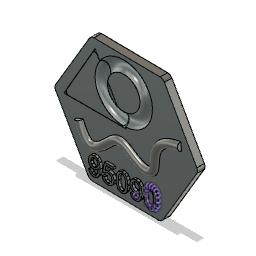
medallion with 95090 Torus Snake v3 (Autodesk Fusion 360 design; units mm, degrees)
Autodesk Fusion 360 part; units mm, degrees
note: some values were not read from the file. Set by a fixed rule: which sketch regions a step uses.
sketch "Sketch1" plane through (0, 0, 0) normal (0, 0, 1) x (1, 0, 0)
  line L0 (13.5687, 24.844) -> (-12.9876, 25.1527)
  line L1 (-14.7311, 24.1729) -> (-28.2766, 1.3288)
  line L2 (-28.2999, -0.6711) -> (-15.2891, -23.8239)
  line L3 (-13.5687, -24.844) -> (12.9876, -25.1527)
  line L4 (14.7311, -24.1729) -> (28.2766, -1.3288)
  line L5 (28.2999, 0.6711) -> (15.2891, 23.8239)
  arc A0 (-12.9876, 25.1527) -> (-14.7311, 24.1729) centre (-13.0108, 23.1528) ccw
  arc A1 (15.2891, 23.8239) -> (13.5687, 24.844) centre (13.5455, 22.8441) ccw
  arc A2 (28.2766, -1.3288) -> (28.2999, 0.6711) centre (26.5563, -0.3087) ccw
  arc A3 (12.9876, -25.1527) -> (14.7311, -24.1729) centre (13.0108, -23.1528) ccw
  arc A4 (-15.2891, -23.8239) -> (-13.5687, -24.844) centre (-13.5455, -22.8441) ccw
  arc A5 (-28.2766, 1.3288) -> (-28.2999, -0.6711) centre (-26.5563, 0.3087) ccw
  point P0 (-12.5, 7.2169)
  dimension "d1" = 25
  dimension "d7" = 2
  dimension "d8" = 2
  dimension "d9" = 2
  dimension "d10" = 2
  dimension "d11" = 2
  dimension "d12" = 2
  constraint tangent L0 A0
  constraint tangent L1 A0
  constraint tangent L0 A1
  constraint tangent L5 A1
  constraint tangent L4 A2
  constraint tangent L5 A2
  constraint tangent L3 A3
  constraint tangent L4 A3
  constraint tangent L2 A4
  constraint tangent L3 A4
  constraint tangent L1 A5
  constraint tangent L2 A5
  measures "d1" distance of origin L5
  measures "d7" radius of A0
  measures "d8" radius of A1
  measures "d9" radius of A2
  measures "d10" radius of A3
  measures "d11" radius of A4
  measures "d12" radius of A5
extrude "Extrude1" add sketch "Sketch1" along normal blind 3 makes body 1
sketch "Sketch2" plane through (0, 0, 0) normal (0, 0, 1) x (1, 0, 0)
  line L0 (-64.3097, 3.8259) -> (-50.5509, -12.3499)
  line L1 (-48.8472, -12.0378) -> (-41.718, 7.9657)
  line L2 (-42.8402, 9.285) -> (-63.7283, 5.4574)
  arc A0 (-41.718, 7.9657) -> (-42.8402, 9.285) centre (-42.6599, 8.3014) ccw
  arc A1 (-50.5509, -12.3499) -> (-48.8472, -12.0378) centre (-49.7892, -11.702) ccw
  arc A2 (-63.7283, 5.4574) -> (-64.3097, 3.8259) centre (-63.548, 4.4738) ccw
  point P0 (-49.4287, -13.6693)
  point P1 (-41.1365, 9.5972)
  point P2 (-53.3624, 0.343)
  dimension "d15" = 24.7
  dimension "d16" = 1
  dimension "d17" = 1
  dimension "d21" = 60
  dimension "d22" = 60
  dimension "d24" = 1
  constraint coincident P1 L1
  constraint coincident P1 L2
  constraint tangent L1 A0
  constraint tangent L2 A0
  constraint coincident P0 L0
  constraint coincident P0 L1
  constraint tangent L0 A1
  constraint tangent L1 A1
  constraint tangent L0 A2
  constraint tangent L2 A2
  measures "d15" distance of P0 P1
  measures "d16" radius of A0
  measures "d17" radius of A1
  measures "d21" angle of L0 L2
  measures "d22" angle of L0 L1
  measures "d24" radius of A2
extrude "Extrude2" add sketch "Sketch2" along normal blind 3 separate body makes body 2
sketch "Sketch4" plane through (0, 0, 3) normal (0, 0, 1) x (1, 0, 0)
  arc A0 (-28.2766, 1.3288) -> (-28.2999, -0.6711) centre (-26.5563, 0.3087) ccw
  line L0 (-28.2999, -0.6711) -> (-15.2891, -23.8239)
  arc A1 (-15.2891, -23.8239) -> (-13.5687, -24.844) centre (-13.5455, -22.8441) ccw
  line L1 (-13.5687, -24.844) -> (12.9876, -25.1527)
  arc A2 (12.9876, -25.1527) -> (14.7311, -24.1729) centre (13.0108, -23.1528) ccw
  line L2 (14.7311, -24.1729) -> (28.2766, -1.3288)
  arc A3 (28.2766, -1.3288) -> (28.2999, 0.6711) centre (26.5563, -0.3087) ccw
  line L3 (28.2999, 0.6711) -> (15.2891, 23.8239)
  arc A4 (15.2891, 23.8239) -> (13.5687, 24.844) centre (13.5455, 22.8441) ccw
  line L4 (13.5687, 24.844) -> (-12.9876, 25.1527)
  arc A5 (-12.9876, 25.1527) -> (-14.7311, 24.1729) centre (-13.0108, 23.1528) ccw
  line L5 (-14.7311, 24.1729) -> (-28.2766, 1.3288)
  line L6 (-12.5, 21.6506) -> (-25, 0)
  line L7 (-25, 0) -> (0, 0)
  line L8 (0, 0) -> (-12.5, 21.6506)
  point P0 (-12.5, 7.2169)
  dimension "d25" = 25
  constraint coincident L7.end L8.start
  constraint horizontal L7
  measures "d25" distance of L6.start L7.end
extrude "Extrude3" cut sketch "Sketch4" against normal up to surface (3 mm away) contours L6 L7 L8 bodies 1
sketch "Sketch5" plane through (0, 0, 3) normal (0, 0, 1) x (1, 0, 0)
  line L0 (-12.5, 21.6506) -> (0, 0)
  line L1 (0, 0) -> (-25, 0)
  line L2 (-25, 0) -> (-12.5, 21.6506)
  arc A0 (-28.2766, 1.3288) -> (-28.2999, -0.6711) centre (-26.5563, 0.3087) ccw
  line L3 (-28.2999, -0.6711) -> (-15.2891, -23.8239)
  arc A1 (-15.2891, -23.8239) -> (-13.5687, -24.844) centre (-13.5455, -22.8441) ccw
  line L4 (-13.5687, -24.844) -> (12.9876, -25.1527)
  arc A2 (12.9876, -25.1527) -> (14.7311, -24.1729) centre (13.0108, -23.1528) ccw
  line L5 (14.7311, -24.1729) -> (28.2766, -1.3288)
  arc A3 (28.2766, -1.3288) -> (28.2999, 0.6711) centre (26.5563, -0.3087) ccw
  line L6 (28.2999, 0.6711) -> (15.2891, 23.8239)
  arc A4 (15.2891, 23.8239) -> (13.5687, 24.844) centre (13.5455, 22.8441) ccw
  line L7 (13.5687, 24.844) -> (-12.9876, 25.1527)
  arc A5 (-12.9876, 25.1527) -> (-14.7311, 24.1729) centre (-13.0108, 23.1528) ccw
  line L8 (-14.7311, 24.1729) -> (-28.2766, 1.3288)
  line L9 (-14.1937, -22.0754) -> (12.7204, -22.0754) construction
  line L10 (12.7204, -22.0754) -> (12.7204, -12.0754) construction
  line L11 (12.7204, -12.0754) -> (-14.1937, -12.0754) construction
  line L12 (-14.1937, -12.0754) -> (-14.1937, -22.0754) construction
  text T0 "95090" font "Arial" height 10 align ink ink in box 0 x 0 at (-14.1837, -22.0554) x (1, 0) y (0, 1) spacing 1 height is em
  constraint perpendicular L9 L10
  constraint parallel L9 L11
  constraint parallel L10 L12
extrude "Extrude4" add sketch "Sketch5" along normal blind 1 text T0 bodies 1
sketch "Sketch6" plane through (0, 0, 3) normal (0, 0, 1) x (1, 0, 0)
  spline S0 degree 3 poles (3.1161, -18.862) (2.9368, -18.6225) (2.5605, -18.1199) (2.5214, -17.4917) (2.5009, -17.1628) knots 0 0 0 0 0.087808 0.184257 0.184257 0.184257 0.184257
  spline S1 degree 3 poles (2.5009, -17.1628) (2.5222, -16.8233) (2.5631, -16.1742) (2.9541, -15.6567) (3.1405, -15.4099) knots 0 0 0 0 0.099559 0.190304 0.190304 0.190304 0.190304
  spline S2 degree 3 poles (3.1405, -15.4099) (3.3707, -15.2162) (3.8369, -14.824) (4.4444, -14.7721) (4.7519, -14.7458) knots 0 0 0 0 0.087967 0.178131 0.178131 0.178131 0.178131
  spline S3 degree 3 poles (4.7519, -14.7458) (4.9791, -14.7612) (5.4319, -14.792) (5.8287, -15.0121) (6.0263, -15.1218) knots 0 0 0 0 0.067431 0.134333 0.134333 0.134333 0.134333
  spline S4 degree 3 poles (6.0263, -15.1218) (6.2093, -15.2633) (6.5846, -15.5535) (6.7966, -15.9783) (6.9052, -16.196) knots 0 0 0 0 0.068468 0.140401 0.140401 0.140401 0.140401
  spline S5 degree 3 poles (6.9052, -16.196) (6.993, -16.4772) (7.1973, -17.1308) (7.2041, -17.8169) (7.2079, -18.2077) knots 0 0 0 0 0.087942 0.2044 0.2044 0.2044 0.2044
  spline S6 degree 3 poles (7.2079, -18.2077) (7.2023, -18.6215) (7.1923, -19.3637) (6.9966, -20.0788) (6.9101, -20.3952) knots 0 0 0 0 0.123516 0.221554 0.221554 0.221554 0.221554
  spline S7 degree 3 poles (6.9101, -20.3952) (6.8034, -20.6457) (6.5995, -21.1249) (6.2081, -21.4672) (6.0214, -21.6306) knots 0 0 0 0 0.080478 0.153934 0.153934 0.153934 0.153934
  spline S8 degree 3 poles (6.0214, -21.6306) (5.8145, -21.7545) (5.3906, -22.0083) (4.8971, -22.0395) (4.6444, -22.0554) knots 0 0 0 0 0.071242 0.145975 0.145975 0.145975 0.145975
  spline S9 degree 3 poles (4.6444, -22.0554) (4.382, -22.04) (3.8811, -22.0107) (3.4687, -21.7267) (3.2724, -21.5915) knots 0 0 0 0 0.07717 0.147318 0.147318 0.147318 0.147318
  spline S10 degree 3 poles (3.2724, -21.5915) (3.1119, -21.4131) (2.7741, -21.0375) (2.6814, -20.5395) (2.6327, -20.2781) knots 0 0 0 0 0.070582 0.148635 0.148635 0.148635 0.148635
  line L0 (2.6327, -20.2781) -> (3.4774, -20.1999)
  spline S11 degree 3 poles (4.664, -21.3327) (4.7929, -21.3262) (5.042, -21.3134) (5.2646, -21.2013) (5.372, -21.1472) knots 0 0 0 0 0.038246 0.07391 0.07391 0.07391 0.07391
  spline S12 degree 3 poles (5.372, -21.1472) (5.47, -21.0801) (5.6666, -20.9453) (5.8053, -20.7514) (5.8749, -20.654) knots 0 0 0 0 0.035331 0.070924 0.070924 0.070924 0.070924
  spline S13 degree 3 poles (5.8749, -20.654) (5.9391, -20.5337) (6.0813, -20.267) (6.1593, -19.9746) (6.2021, -19.8142) knots 0 0 0 0 0.040781 0.090394 0.090394 0.090394 0.090394
  spline S14 degree 3 poles (6.3339, -18.74) (6.3336, -18.7156) (6.3328, -18.6569) (6.3304, -18.5984) (6.329, -18.5642) knots 0 0 0 0 0.007325 0.017586 0.017586 0.017586 0.017586
  spline S15 degree 3 poles (6.329, -18.5642) (6.2317, -18.6984) (6.0337, -18.9714) (5.7504, -19.1546) (5.6064, -19.2478) knots 0 0 0 0 0.049266 0.100244 0.100244 0.100244 0.100244
  spline S16 degree 3 poles (5.6064, -19.2478) (5.4513, -19.3233) (5.1397, -19.4749) (4.7938, -19.496) (4.62, -19.5066) knots 0 0 0 0 0.051186 0.102862 0.102862 0.102862 0.102862
  arc A0 (-28.2766, 1.3288) -> (-28.2999, -0.6711) centre (-26.5563, 0.3087) ccw
  line L1 (-28.2999, -0.6711) -> (-15.2891, -23.8239)
  arc A1 (-15.2891, -23.8239) -> (-13.5687, -24.844) centre (-13.5455, -22.8441) ccw
  line L2 (-13.5687, -24.844) -> (12.9876, -25.1527)
  arc A2 (12.9876, -25.1527) -> (14.7311, -24.1729) centre (13.0108, -23.1528) ccw
  line L3 (14.7311, -24.1729) -> (28.2766, -1.3288)
  arc A3 (28.2766, -1.3288) -> (28.2999, 0.6711) centre (26.5563, -0.3087) ccw
  line L4 (28.2999, 0.6711) -> (15.2891, 23.8239)
  arc A4 (15.2891, 23.8239) -> (13.5687, 24.844) centre (13.5455, 22.8441) ccw
  line L5 (13.5687, 24.844) -> (-12.9876, 25.1527)
  arc A5 (-12.9876, 25.1527) -> (-14.7311, 24.1729) centre (-13.0108, 23.1528) ccw
  line L6 (-14.7311, 24.1729) -> (-28.2766, 1.3288)
  line L7 (-12.5, 21.6506) -> (0, 0)
  line L8 (0, 0) -> (-25, 0)
  line L9 (-25, 0) -> (-12.5, 21.6506)
  line L10 (-8.6222, -20.0583) -> (-7.6993, -19.9802)
  spline S17 degree 3 poles (-7.6993, -19.9802) (-7.6597, -20.1853) (-7.5864, -20.5648) (-7.3392, -20.8601) (-7.2257, -20.9958) knots 0 0 0 0 0.06147 0.113705 0.113705 0.113705 0.113705
  spline S18 degree 3 poles (-7.2257, -20.9958) (-7.093, -21.0941) (-6.8244, -21.293) (-6.4911, -21.3194) (-6.3224, -21.3327) knots 0 0 0 0 0.048487 0.098156 0.098156 0.098156 0.098156
  spline S19 degree 3 poles (-6.3224, -21.3327) (-6.1184, -21.3123) (-5.7079, -21.2711) (-5.4021, -20.9938) (-5.2481, -20.8542) knots 0 0 0 0 0.059802 0.120401 0.120401 0.120401 0.120401
  spline S20 degree 3 poles (-5.2481, -20.8542) (-5.1201, -20.6752) (-4.8492, -20.2965) (-4.8227, -19.8304) (-4.8087, -19.5847) knots 0 0 0 0 0.06469 0.136821 0.136821 0.136821 0.136821
  spline S21 degree 3 poles (-4.8087, -19.5847) (-4.8218, -19.3522) (-4.8465, -18.9133) (-5.1097, -18.5629) (-5.2335, -18.3982) knots 0 0 0 0 0.068094 0.12856 0.12856 0.12856 0.12856
  spline S22 degree 3 poles (-5.2335, -18.3982) (-5.3882, -18.2715) (-5.7087, -18.0089) (-6.1228, -17.9791) (-6.337, -17.9636) knots 0 0 0 0 0.058504 0.12122 0.12122 0.12122 0.12122
  spline S23 degree 3 poles (-6.337, -17.9636) (-6.474, -17.9711) (-6.7425, -17.9857) (-6.9849, -18.102) (-7.1036, -18.1589) knots 0 0 0 0 0.040699 0.079802 0.079802 0.079802 0.079802
  spline S24 degree 3 poles (-7.1036, -18.1589) (-7.2108, -18.2263) (-7.4213, -18.3586) (-7.5685, -18.5587) (-7.6407, -18.657) knots 0 0 0 0 0.037605 0.073834 0.073834 0.073834 0.073834
  line L11 (-7.6407, -18.657) -> (-8.4659, -18.5495)
  line L12 (-8.4659, -18.5495) -> (-7.7726, -14.8728)
  line L13 (-7.7726, -14.8728) -> (-4.213, -14.8728)
  line L14 (-4.213, -14.8728) -> (-4.213, -15.7126)
  line L15 (-4.213, -15.7126) -> (-7.0694, -15.7126)
  line L16 (-7.0694, -15.7126) -> (-7.4552, -17.6365)
  spline S25 degree 3 poles (-7.4552, -17.6365) (-7.2412, -17.5055) (-6.8247, -17.2506) (-6.3388, -17.208) (-6.1026, -17.1872) knots 0 0 0 0 0.074138 0.144257 0.144257 0.144257 0.144257
  spline S26 degree 3 poles (-6.1026, -17.1872) (-5.8031, -17.2135) (-5.2081, -17.2658) (-4.7487, -17.6472) (-4.5206, -17.8367) knots 0 0 0 0 0.087937 0.17468 0.17468 0.17468 0.17468
  spline S27 degree 3 poles (-4.5206, -17.8367) (-4.3327, -18.0735) (-3.9449, -18.5622) (-3.8995, -19.1854) (-3.8761, -19.5066) knots 0 0 0 0 0.088573 0.182735 0.182735 0.182735 0.182735
  spline S28 degree 3 poles (-3.8761, -19.5066) (-3.8978, -19.8172) (-3.9406, -20.4269) (-4.2773, -20.9363) (-4.4425, -21.1863) knots 0 0 0 0 0.091676 0.179961 0.179961 0.179961 0.179961
  spline S29 degree 3 poles (-4.4425, -21.1863) (-4.6969, -21.4397) (-5.2167, -21.9575) (-5.9487, -22.0223) (-6.3224, -22.0554) knots 0 0 0 0 0.1043 0.21306 0.21306 0.21306 0.21306
  spline S30 degree 3 poles (-6.3224, -22.0554) (-6.6278, -22.0371) (-7.2119, -22.0021) (-7.6906, -21.6679) (-7.919, -21.5085) knots 0 0 0 0 0.089792 0.171721 0.171721 0.171721 0.171721
  spline S31 degree 3 poles (-7.919, -21.5085) (-8.1025, -21.3075) (-8.4796, -20.8942) (-8.5738, -20.342) (-8.6222, -20.0583) knots 0 0 0 0 0.079884 0.164218 0.164218 0.164218 0.164218
  spline S32 degree 3 poles (-3.0606, -18.4031) (-3.0556, -18.0191) (-3.0464, -17.3283) (-2.8771, -16.6593) (-2.8018, -16.362) knots 0 0 0 0 0.114685 0.206362 0.206362 0.206362 0.206362
  spline S33 degree 3 poles (-2.8018, -16.362) (-2.7089, -16.1226) (-2.5328, -15.6692) (-2.1881, -15.3272) (-2.0255, -15.1658) knots 0 0 0 0 0.076062 0.144034 0.144034 0.144034 0.144034
  spline S34 degree 3 poles (-2.0255, -15.1658) (-1.8368, -15.0433) (-1.4423, -14.7874) (-0.972, -14.7601) (-0.7267, -14.7458) knots 0 0 0 0 0.066307 0.138606 0.138606 0.138606 0.138606
  spline S35 degree 3 poles (-0.7267, -14.7458) (-0.5437, -14.7539) (-0.1919, -14.7695) (0.1297, -14.9119) (0.2841, -14.9802) knots 0 0 0 0 0.054394 0.10457 0.10457 0.10457 0.10457
  spline S36 degree 3 poles (0.2841, -14.9802) (0.4234, -15.0666) (0.7066, -15.2423) (0.9024, -15.5121) (1.0019, -15.6492) knots 0 0 0 0 0.048673 0.098953 0.098953 0.098953 0.098953
  spline S37 degree 3 poles (1.0019, -15.6492) (1.0925, -15.8076) (1.2849, -16.1437) (1.3904, -16.5165) (1.4462, -16.7136) knots 0 0 0 0 0.054546 0.11573 0.11573 0.11573 0.11573
  spline S38 degree 3 poles (1.4462, -16.7136) (1.493, -16.9579) (1.5999, -17.5156) (1.6047, -18.0838) (1.6073, -18.4031) knots 0 0 0 0 0.074473 0.170017 0.170017 0.170017 0.170017
  spline S39 degree 3 poles (1.6073, -18.4031) (1.6021, -18.7849) (1.5926, -19.474) (1.4238, -20.1415) (1.3485, -20.4392) knots 0 0 0 0 0.114075 0.205872 0.205872 0.205872 0.205872
  spline S40 degree 3 poles (1.3485, -20.4392) (1.2564, -20.6778) (1.081, -21.1316) (0.7359, -21.4734) (0.5722, -21.6355) knots 0 0 0 0 0.075737 0.144053 0.144053 0.144053 0.144053
  spline S41 degree 3 poles (0.5722, -21.6355) (0.3843, -21.7579) (-0.0098, -22.0146) (-0.4804, -22.0414) (-0.7267, -22.0554) knots 0 0 0 0 0.066092 0.138633 0.138633 0.138633 0.138633
  spline S42 degree 3 poles (-0.7267, -22.0554) (-1.0505, -22.0277) (-1.6823, -21.9738) (-2.133, -21.5296) (-2.3526, -21.3132) knots 0 0 0 0 0.094252 0.183835 0.183835 0.183835 0.183835
  spline S43 degree 3 poles (-2.3526, -21.3132) (-2.558, -20.9294) (-3.0413, -20.026) (-3.0536, -18.9957) (-3.0606, -18.4031) knots 0 0 0 0 0.128879 0.303363 0.303363 0.303363 0.303363
  line L17 (-14.0518, -20.2781) -> (-13.2071, -20.1999)
  spline S44 degree 3 poles (-13.2071, -20.1999) (-13.1697, -20.3785) (-13.1022, -20.701) (-12.8911, -20.9521) (-12.797, -21.0642) knots 0 0 0 0 0.053714 0.096982 0.096982 0.096982 0.096982
  spline S45 degree 3 poles (-12.797, -21.0642) (-12.6858, -21.1425) (-12.4533, -21.3061) (-12.1689, -21.3236) (-12.0206, -21.3327) knots 0 0 0 0 0.039989 0.0836 0.0836 0.0836 0.0836
  spline S46 degree 3 poles (-12.0206, -21.3327) (-11.8917, -21.3262) (-11.6426, -21.3134) (-11.42, -21.2013) (-11.3126, -21.1472) knots 0 0 0 0 0.038246 0.07391 0.07391 0.07391 0.07391
  spline S47 degree 3 poles (-11.3126, -21.1472) (-11.2146, -21.0801) (-11.0179, -20.9453) (-10.8793, -20.7514) (-10.8097, -20.654) knots 0 0 0 0 0.035331 0.070924 0.070924 0.070924 0.070924
  spline S48 degree 3 poles (-10.8097, -20.654) (-10.7455, -20.5337) (-10.6032, -20.267) (-10.5253, -19.9746) (-10.4825, -19.8142) knots 0 0 0 0 0.040781 0.090394 0.090394 0.090394 0.090394
  spline S49 degree 3 poles (-10.4825, -19.8142) (-10.4441, -19.6375) (-10.367, -19.2834) (-10.3561, -18.9213) (-10.3507, -18.74) knots 0 0 0 0 0.054133 0.108433 0.108433 0.108433 0.108433
  spline S50 degree 3 poles (-10.3507, -18.74) (-10.351, -18.7156) (-10.3517, -18.6569) (-10.3541, -18.5984) (-10.3556, -18.5642) knots 0 0 0 0 0.007325 0.017586 0.017586 0.017586 0.017586
  spline S51 degree 3 poles (-10.3556, -18.5642) (-10.4529, -18.6984) (-10.6508, -18.9714) (-10.9341, -19.1546) (-11.0782, -19.2478) knots 0 0 0 0 0.049266 0.100244 0.100244 0.100244 0.100244
  spline S52 degree 3 poles (-11.0782, -19.2478) (-11.2333, -19.3233) (-11.5448, -19.4749) (-11.8908, -19.496) (-12.0645, -19.5066) knots 0 0 0 0 0.051186 0.102862 0.102862 0.102862 0.102862
  spline S53 degree 3 poles (-12.0645, -19.5066) (-12.3495, -19.4796) (-12.9197, -19.4257) (-13.3521, -19.05) (-13.5685, -18.862) knots 0 0 0 0 0.083599 0.167323 0.167323 0.167323 0.167323
  spline S54 degree 3 poles (-13.5685, -18.862) (-13.7478, -18.6225) (-14.1241, -18.1199) (-14.1632, -17.4917) (-14.1837, -17.1628) knots 0 0 0 0 0.087808 0.184257 0.184257 0.184257 0.184257
  spline S55 degree 3 poles (-14.1837, -17.1628) (-14.1623, -16.8233) (-14.1215, -16.1742) (-13.7305, -15.6567) (-13.544, -15.4099) knots 0 0 0 0 0.099559 0.190304 0.190304 0.190304 0.190304
  spline S56 degree 3 poles (-13.544, -15.4099) (-13.3138, -15.2162) (-12.8476, -14.824) (-12.2402, -14.7721) (-11.9327, -14.7458) knots 0 0 0 0 0.087967 0.178131 0.178131 0.178131 0.178131
  spline S57 degree 3 poles (-11.9327, -14.7458) (-11.7054, -14.7612) (-11.2527, -14.792) (-10.8559, -15.0121) (-10.6583, -15.1218) knots 0 0 0 0 0.067431 0.134333 0.134333 0.134333 0.134333
  spline S58 degree 3 poles (-10.6583, -15.1218) (-10.4753, -15.2633) (-10.0999, -15.5535) (-9.888, -15.9783) (-9.7794, -16.196) knots 0 0 0 0 0.068468 0.140401 0.140401 0.140401 0.140401
  spline S59 degree 3 poles (-9.7794, -16.196) (-9.6915, -16.4772) (-9.4873, -17.1308) (-9.4805, -17.8169) (-9.4767, -18.2077) knots 0 0 0 0 0.087942 0.2044 0.2044 0.2044 0.2044
  spline S60 degree 3 poles (-9.4767, -18.2077) (-9.4822, -18.6215) (-9.4923, -19.3637) (-9.6879, -20.0788) (-9.7745, -20.3952) knots 0 0 0 0 0.123516 0.221554 0.221554 0.221554 0.221554
  spline S61 degree 3 poles (-9.7745, -20.3952) (-9.8811, -20.6457) (-10.0851, -21.1249) (-10.4764, -21.4672) (-10.6632, -21.6306) knots 0 0 0 0 0.080478 0.153934 0.153934 0.153934 0.153934
  spline S62 degree 3 poles (-10.6632, -21.6306) (-10.87, -21.7545) (-11.2939, -22.0083) (-11.7875, -22.0395) (-12.0401, -22.0554) knots 0 0 0 0 0.071242 0.145975 0.145975 0.145975 0.145975
  spline S63 degree 3 poles (-12.0401, -22.0554) (-12.3025, -22.04) (-12.8035, -22.0107) (-13.2159, -21.7267) (-13.4122, -21.5915) knots 0 0 0 0 0.07717 0.147318 0.147318 0.147318 0.147318
  spline S64 degree 3 poles (-13.4122, -21.5915) (-13.5726, -21.4131) (-13.9105, -21.0375) (-14.0032, -20.5395) (-14.0518, -20.2781) knots 0 0 0 0 0.070582 0.148635 0.148635 0.148635 0.148635
  spline S65 degree 3 poles (8.0624, -18.4031) (8.0675, -18.0191) (8.0766, -17.3283) (8.246, -16.6593) (8.3212, -16.362) knots 0 0 0 0 0.114685 0.206362 0.206362 0.206362 0.206362
  spline S66 degree 3 poles (8.3212, -16.362) (8.4142, -16.1226) (8.5902, -15.6692) (8.9349, -15.3272) (9.0976, -15.1658) knots 0 0 0 0 0.076062 0.144034 0.144034 0.144034 0.144034
  spline S67 degree 3 poles (9.0976, -15.1658) (9.2863, -15.0433) (9.6808, -14.7874) (10.1511, -14.7601) (10.3964, -14.7458) knots 0 0 0 0 0.066307 0.138606 0.138606 0.138606 0.138606
  spline S68 degree 3 poles (10.3964, -14.7458) (10.5794, -14.7539) (10.9311, -14.7695) (11.2528, -14.9119) (11.4071, -14.9802) knots 0 0 0 0 0.054394 0.10457 0.10457 0.10457 0.10457
  spline S69 degree 3 poles (11.4071, -14.9802) (11.5464, -15.0666) (11.8296, -15.2423) (12.0254, -15.5121) (12.1249, -15.6492) knots 0 0 0 0 0.048673 0.098953 0.098953 0.098953 0.098953
  spline S70 degree 3 poles (12.1249, -15.6492) (12.2156, -15.8076) (12.4079, -16.1437) (12.5134, -16.5165) (12.5692, -16.7136) knots 0 0 0 0 0.054546 0.11573 0.11573 0.11573 0.11573
  spline S71 degree 3 poles (12.5692, -16.7136) (12.6161, -16.9579) (12.7229, -17.5156) (12.7277, -18.0838) (12.7304, -18.4031) knots 0 0 0 0 0.074473 0.170017 0.170017 0.170017 0.170017
  spline S72 degree 3 poles (12.7304, -18.4031) (12.7251, -18.7849) (12.7156, -19.474) (12.5468, -20.1415) (12.4716, -20.4392) knots 0 0 0 0 0.114075 0.205872 0.205872 0.205872 0.205872
  spline S73 degree 3 poles (12.4716, -20.4392) (12.3794, -20.6778) (12.2041, -21.1316) (11.8589, -21.4734) (11.6952, -21.6355) knots 0 0 0 0 0.075737 0.144053 0.144053 0.144053 0.144053
  spline S74 degree 3 poles (11.6952, -21.6355) (11.5073, -21.7579) (11.1132, -22.0146) (10.6426, -22.0414) (10.3964, -22.0554) knots 0 0 0 0 0.066092 0.138633 0.138633 0.138633 0.138633
  spline S75 degree 3 poles (10.3964, -22.0554) (10.0725, -22.0277) (9.4408, -21.9738) (8.9901, -21.5296) (8.7704, -21.3132) knots 0 0 0 0 0.094252 0.183835 0.183835 0.183835 0.183835
  spline S76 degree 3 poles (8.7704, -21.3132) (8.5651, -20.9294) (8.0817, -20.026) (8.0695, -18.9957) (8.0624, -18.4031) knots 0 0 0 0 0.128879 0.303363 0.303363 0.303363 0.303363
  spline S77 degree 3 poles (3.4774, -20.1999) (3.5149, -20.3785) (3.5824, -20.701) (3.7934, -20.9521) (3.8876, -21.0642) knots 0 0 0 0 0.053714 0.096982 0.096982 0.096982 0.096982
  spline S78 degree 3 poles (3.8876, -21.0642) (3.9988, -21.1425) (4.2313, -21.3061) (4.5156, -21.3236) (4.664, -21.3327) knots 0 0 0 0 0.039989 0.0836 0.0836 0.0836 0.0836
  spline S79 degree 3 poles (6.2021, -19.8142) (6.2405, -19.6375) (6.3175, -19.2834) (6.3284, -18.9213) (6.3339, -18.74) knots 0 0 0 0 0.054133 0.108433 0.108433 0.108433 0.108433
  spline S80 degree 3 poles (4.62, -19.5066) (4.3351, -19.4796) (3.7649, -19.4257) (3.3325, -19.05) (3.1161, -18.862) knots 0 0 0 0 0.083599 0.167323 0.167323 0.167323 0.167323
move_body "Move1" bodies 2 to x (0.337095, -0.941471, 0) y (0.941471, 0.337095, 0) z (0, 0, 1) at (4.6751, -41.8673, 0)
torus "TorusPrimitive1" cut centre line diameter 18 section diameter 5 placed x (1, 0, 0) y (0, 1, 0) z (0, 0, 1) at (-1, 12, 3) bodies 1 2
sketch "Sketch10" plane through (0, 0, 3) normal (0, 0, 1) x (1, 0, 0)
  spline S0 degree 5 poles (-18.6017, -5.6454) (-18.3665, -6.2766) (-17.8901, -7.4615) (-17.1577, -9.0061) (-16.1454, -10.5996) (-14.8212, -11.8215) (-13.4413, -12.2999) (-12.0126, -12.093) (-10.5465, -11.3011) (-9.0609, -10.0831) (-7.579, -8.6499) (-6.1232, -7.2299) (-4.7102, -6.0415) (-3.3451, -5.2617) (-2.0179, -4.9997) (-0.6948, -5.259) (0.672, -5.9468) (2.1257, -6.9098) (3.6871, -7.962) (5.3399, -8.9144) (7.0064, -9.6066) (8.5602, -9.9234) (9.869, -9.7943) (10.8301, -9.1992) (11.4079, -8.1713) (11.6729, -6.8022) (11.7638, -5.2194) (11.8461, -3.5621) (12.0753, -1.9596) (12.5525, -0.5056) (13.298, 0.7576) (14.2805, 1.8222) (15.4378, 2.7031) (16.6988, 3.4253) (18.0095, 4.0097) (19.3388, 4.468) (20.4045, 4.7393) (21.2026, 4.8901) (21.7343, 4.9672) (22, 5) knots 0 0 0 0 0 0 0.028571 0.057143 0.085714 0.114286 0.142857 0.171429 0.2 0.228571 0.257143 0.285714 0.314286 0.342857 0.371429 0.4 0.428571 0.457143 0.485714 0.514286 0.542857 0.571429 0.6 0.628571 0.657143 0.685714 0.714286 0.742857 0.771429 0.8 0.828571 0.857143 0.885714 0.914286 0.942857 0.971429 1 1 1 1 1 1
  point P0 (-11.2104, -11.5994)
  point P1 (-2.8611, -5.2347)
  point P2 (4.4617, -8.3829)
  point P3 (10.758, -9.0672)
  point P4 (12.0583, -2.3604)
  point P5 (16, 3)
pipe "Pipe1" add diameter 3 path "Sketch10" along S0 bodies 1
